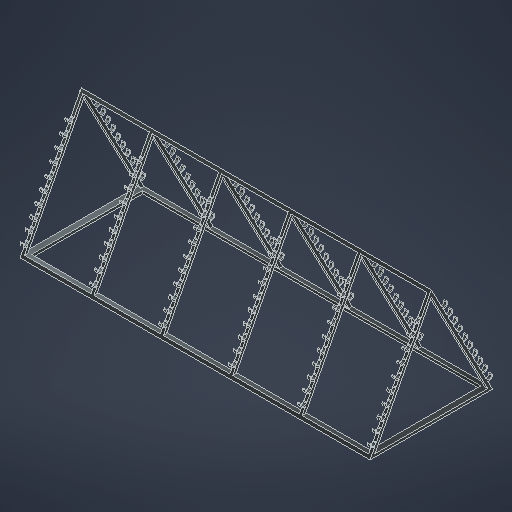
# Autodesk Inventor part: Torre
Saved by Autodesk Inventor 2026.1 (Build 301233020, 233B)
## iProperties
Created: 2025-11-02
Part Number: Torre
Material: Hierro, gris
Document SubType Name: Modeling
Designer: PAVILION
Density: 7.15 g/cm^3
Appearance: Gris hierro
Author: PAVILION
Autodesk Inventor part; units mm, degrees
ref_plane "YZ Plane" through (0, 0, 0) normal (1, 0, 0) x (0, 1, 0)
ref_plane "XZ Plane" through (0, 0, 0) normal (0, 1, 0) x (-1, 0, 0)
ref_plane "XY Plane" through (0, 0, 0) normal (0, 0, 1) x (1, 0, 0)
sketch "Boceto2" plane through (0, 0, 0) normal (1, 0, 0) x (0, 1, 0)
  line L0 (0, 0) -> (2000, 0)
  line L1 (0, 1050) -> (0, -1050)
  line L2 (2000, 0) -> (0, 1050)
  line L3 (2000, 0) -> (0, -1050)
  line L4 (1892.4347, 0) -> (50, 967.2782)
  line L5 (50, 967.2782) -> (50, -967.2782)
  line L6 (50, -967.2782) -> (1892.4347, 0)
  line L7 (200, 945) -> (200, -945)
  line L8 (362, 859.95) -> (362, -859.95)
  line L9 (524, 774.9) -> (524, -774.9)
  line L10 (686, 689.85) -> (686, -689.85)
  line L11 (848, 604.8) -> (848, -604.8)
  line L12 (1010, 519.75) -> (1010, -519.75)
  line L13 (1172, 434.7) -> (1172, -434.7)
  line L14 (1334, 349.65) -> (1334, -349.65)
  line L15 (1496, 264.6) -> (1496, -264.6)
  line L16 (1658, 179.55) -> (1658, -179.55)
  arc A0 (222.9629, 1038.4173) -> (200, 945) centre (211.77, 991.6377) ccw construction
  arc A1 (225.2899, 1048.1428) -> (197.553, 935.304) centre (211.77, 991.6377) ccw
  arc A2 (220.6359, 1028.6918) -> (202.447, 954.696) centre (211.77, 991.6377) ccw
  arc A3 (220.6359, 1028.6918) -> (225.2899, 1048.1428) centre (222.9629, 1038.4173) ccw
  arc A4 (197.553, 935.304) -> (202.447, 954.696) centre (200, 945) ccw
  arc A5 (388.0719, 952.4704) -> (362, 859.95) centre (376.879, 905.6908) ccw construction
  arc A6 (390.3989, 962.1959) -> (358.9066, 850.4405) centre (376.879, 905.6908) ccw
  arc A7 (385.7449, 942.7449) -> (365.0934, 869.4595) centre (376.879, 905.6908) ccw
  arc A8 (385.7449, 942.7449) -> (390.3989, 962.1959) centre (388.0719, 952.4704) ccw
  arc A9 (358.9066, 850.4405) -> (365.0934, 869.4595) centre (362, 859.95) ccw
  arc A10 (524.6943, 764.9241) -> (523.3057, 784.8759) centre (524, 774.9) ccw
  arc A11 (538.8131, 856.3817) -> (548.3419, 873.9658) centre (543.5775, 865.1737) ccw
  arc A12 (538.8131, 856.3817) -> (523.3057, 784.8759) centre (520.6606, 822.8839) ccw
  arc A13 (543.5775, 865.1737) -> (524, 774.9) centre (520.6606, 822.8839) ccw construction
  arc A14 (548.3419, 873.9658) -> (524.6943, 764.9241) centre (520.6606, 822.8839) ccw
  arc A15 (686.078, 679.8503) -> (685.922, 699.8497) centre (686, 689.85) ccw
  arc A16 (695.4303, 774.7651) -> (700.5775, 794.0915) centre (698.0039, 784.4283) ccw
  arc A17 (695.4303, 774.7651) -> (685.922, 699.8497) centre (685.6249, 737.9485) ccw
  arc A18 (698.0039, 784.4283) -> (686, 689.85) centre (685.6249, 737.9485) ccw construction
  arc A19 (700.5775, 794.0915) -> (686.078, 679.8503) centre (685.6249, 737.9485) ccw
  arc A20 (848.9573, 594.8459) -> (847.0427, 614.7541) centre (848, 604.8) ccw
  arc A21 (855.7302, 688.7271) -> (862.2053, 707.6499) centre (858.9678, 698.1885) ccw
  arc A22 (858.9678, 698.1885) -> (848, 604.8) centre (843.3952, 652.6791) ccw construction
  arc A23 (862.2053, 707.6499) -> (848.9573, 594.8459) centre (843.3952, 652.6791) ccw
  arc A24 (855.7302, 688.7271) -> (847.0427, 614.7541) centre (843.3952, 652.6791) ccw
  arc A25 (1010.4664, 509.7609) -> (1009.5336, 529.7391) centre (1010, 519.75) ccw
  arc A26 (1014.5671, 605.284) -> (1018.1422, 624.9619) centre (1016.3547, 615.1229) ccw
  arc A27 (1014.5671, 605.284) -> (1009.5336, 529.7391) centre (1007.7565, 567.7976) ccw
  arc A28 (1016.3547, 615.1229) -> (1010, 519.75) centre (1007.7565, 567.7976) ccw construction
  arc A29 (1018.1422, 624.9619) -> (1010.4664, 509.7609) centre (1007.7565, 567.7976) ccw
  arc A30 (1170.3484, 424.8373) -> (1173.6516, 444.5627) centre (1172, 434.7) ccw
  arc A31 (1185.089, 519.8905) -> (1173.6516, 444.5627) centre (1179.9441, 482.1395) ccw
  arc A32 (1186.4394, 529.7989) -> (1172, 434.7) centre (1179.9441, 482.1395) ccw construction
  arc A33 (1187.7898, 539.7073) -> (1170.3484, 424.8373) centre (1179.9441, 482.1395) ccw
  arc A34 (1185.089, 519.8905) -> (1187.7898, 539.7073) centre (1186.4394, 529.7989) ccw
  arc A35 (1331.7811, 339.8993) -> (1336.2189, 359.4007) centre (1334, 349.65) ccw
  arc A36 (1351.0826, 434.1079) -> (1336.2189, 359.4007) centre (1344.6731, 396.5509) ccw
  arc A37 (1352.7649, 443.9654) -> (1334, 349.65) centre (1344.6731, 396.5509) ccw construction
  arc A38 (1354.4472, 453.8229) -> (1331.7811, 339.8993) centre (1344.6731, 396.5509) ccw
  arc A39 (1351.0826, 434.1079) -> (1354.4472, 453.8229) centre (1352.7649, 443.9654) ccw
  arc A40 (1517.4545, 348.081) -> (1522.6924, 367.383) centre (1520.0734, 357.732) ccw
  arc A41 (1517.4545, 348.081) -> (1498.386, 274.3112) centre (1507.4764, 311.3108) ccw
  arc A42 (1493.614, 254.8888) -> (1498.386, 274.3112) centre (1496, 264.6) ccw
  arc A43 (1520.0734, 357.732) -> (1496, 264.6) centre (1507.4764, 311.3108) ccw construction
  arc A44 (1522.6924, 367.383) -> (1493.614, 254.8888) centre (1507.4764, 311.3108) ccw
  arc A45 (1654.6752, 170.1189) -> (1661.3248, 188.9811) centre (1658, 179.55) ccw
  arc A46 (1683.3502, 261.8465) -> (1661.3248, 188.9811) centre (1673.9925, 224.9135) ccw
  arc A47 (1685.8063, 271.5402) -> (1658, 179.55) centre (1673.9925, 224.9135) ccw construction
  arc A48 (1688.2623, 281.2339) -> (1654.6752, 170.1189) centre (1673.9925, 224.9135) ccw
  arc A49 (1683.3502, 261.8465) -> (1688.2623, 281.2339) centre (1685.8063, 271.5402) ccw
  arc A50 (200, -945) -> (222.9629, -1038.4173) centre (211.77, -991.6377) ccw construction
  arc A51 (197.553, -935.304) -> (225.2899, -1048.1428) centre (211.77, -991.6377) ccw
  arc A52 (202.447, -954.696) -> (220.6359, -1028.6918) centre (211.77, -991.6377) ccw
  arc A53 (225.2899, -1048.1428) -> (220.6359, -1028.6918) centre (222.9629, -1038.4173) ccw
  arc A54 (202.447, -954.696) -> (197.553, -935.304) centre (200, -945) ccw
  arc A55 (365.0934, -869.4595) -> (358.9066, -850.4405) centre (362, -859.95) ccw
  arc A56 (390.3989, -962.1959) -> (385.7449, -942.7449) centre (388.0719, -952.4704) ccw
  arc A57 (365.0934, -869.4595) -> (385.7449, -942.7449) centre (376.879, -905.6908) ccw
  arc A58 (362, -859.95) -> (388.0719, -952.4704) centre (376.879, -905.6908) ccw construction
  arc A59 (358.9066, -850.4405) -> (390.3989, -962.1959) centre (376.879, -905.6908) ccw
  arc A60 (523.3057, -784.8759) -> (524.6943, -764.9241) centre (524, -774.9) ccw
  arc A61 (548.3419, -873.9658) -> (538.8131, -856.3817) centre (543.5775, -865.1737) ccw
  arc A62 (523.3057, -784.8759) -> (538.8131, -856.3817) centre (520.6606, -822.8839) ccw
  arc A63 (524, -774.9) -> (543.5775, -865.1737) centre (520.6606, -822.8839) ccw construction
  arc A64 (524.6943, -764.9241) -> (548.3419, -873.9658) centre (520.6606, -822.8839) ccw
  arc A65 (685.922, -699.8497) -> (686.078, -679.8503) centre (686, -689.85) ccw
  arc A66 (700.5775, -794.0915) -> (695.4303, -774.7651) centre (698.0039, -784.4283) ccw
  arc A67 (686, -689.85) -> (698.0039, -784.4283) centre (685.6249, -737.9485) ccw construction
  arc A68 (686.078, -679.8503) -> (700.5775, -794.0915) centre (685.6249, -737.9485) ccw
  arc A69 (685.922, -699.8497) -> (695.4303, -774.7651) centre (685.6249, -737.9485) ccw
  arc A70 (847.0427, -614.7541) -> (848.9573, -594.8459) centre (848, -604.8) ccw
  arc A71 (862.2053, -707.6499) -> (855.7302, -688.7271) centre (858.9678, -698.1885) ccw
  arc A72 (847.0427, -614.7541) -> (855.7302, -688.7271) centre (843.3952, -652.6791) ccw
  arc A73 (848, -604.8) -> (858.9678, -698.1885) centre (843.3952, -652.6791) ccw construction
  arc A74 (848.9573, -594.8459) -> (862.2053, -707.6499) centre (843.3952, -652.6791) ccw
  arc A75 (1009.5336, -529.7391) -> (1010.4664, -509.7609) centre (1010, -519.75) ccw
  arc A76 (1009.5336, -529.7391) -> (1014.5671, -605.284) centre (1007.7565, -567.7976) ccw
  arc A77 (1010, -519.75) -> (1016.3547, -615.1229) centre (1007.7565, -567.7976) ccw construction
  arc A78 (1010.4664, -509.7609) -> (1018.1422, -624.9619) centre (1007.7565, -567.7976) ccw
  arc A79 (1018.1422, -624.9619) -> (1014.5671, -605.284) centre (1016.3547, -615.1229) ccw
  arc A80 (1173.6516, -444.5627) -> (1170.3484, -424.8373) centre (1172, -434.7) ccw
  arc A81 (1173.6516, -444.5627) -> (1185.089, -519.8905) centre (1179.9441, -482.1395) ccw
  arc A82 (1172, -434.7) -> (1186.4394, -529.7989) centre (1179.9441, -482.1395) ccw construction
  arc A83 (1170.3484, -424.8373) -> (1187.7898, -539.7073) centre (1179.9441, -482.1395) ccw
  arc A84 (1187.7898, -539.7073) -> (1185.089, -519.8905) centre (1186.4394, -529.7989) ccw
  arc A85 (1354.4472, -453.8229) -> (1351.0826, -434.1079) centre (1352.7649, -443.9654) ccw
  arc A86 (1336.2189, -359.4007) -> (1351.0826, -434.1079) centre (1344.6731, -396.5509) ccw
  arc A87 (1336.2189, -359.4007) -> (1331.7811, -339.8993) centre (1334, -349.65) ccw
  arc A88 (1334, -349.65) -> (1352.7649, -443.9654) centre (1344.6731, -396.5509) ccw construction
  arc A89 (1331.7811, -339.8993) -> (1354.4472, -453.8229) centre (1344.6731, -396.5509) ccw
  arc A90 (1498.386, -274.3112) -> (1493.614, -254.8888) centre (1496, -264.6) ccw
  arc A91 (1498.386, -274.3112) -> (1517.4545, -348.081) centre (1507.4764, -311.3108) ccw
  arc A92 (1496, -264.6) -> (1520.0734, -357.732) centre (1507.4764, -311.3108) ccw construction
  arc A93 (1493.614, -254.8888) -> (1522.6924, -367.383) centre (1507.4764, -311.3108) ccw
  arc A94 (1522.6924, -367.383) -> (1517.4545, -348.081) centre (1520.0734, -357.732) ccw
  arc A95 (1688.2623, -281.2339) -> (1683.3502, -261.8465) centre (1685.8063, -271.5402) ccw
  arc A96 (1654.6752, -170.1189) -> (1688.2623, -281.2339) centre (1673.9925, -224.9135) ccw
  arc A97 (1661.3248, -188.9811) -> (1683.3502, -261.8465) centre (1673.9925, -224.9135) ccw
  arc A98 (1658, -179.55) -> (1685.8063, -271.5402) centre (1673.9925, -224.9135) ccw construction
  arc A99 (1661.3248, -188.9811) -> (1654.6752, -170.1189) centre (1658, -179.55) ccw
  point P0 (362, 0)
  point P1 (312.784, 788.7029)
  point P2 (524, 0)
  point P3 (461.0296, 697.0924)
  point P4 (686, 0)
  point P5 (835.0047, 590.2711)
  point P6 (848, 0)
  point P7 (804.8988, 519.75)
  point P8 (788.1671, 504.3238)
  point P9 (1010, 0)
  point P10 (971.3706, 434.7)
  point P11 (1172, 0)
  point P12 (1199.0684, 349.65)
  point P13 (1334, 0)
  point P14 (1280.8287, 264.6)
  point P15 (1496, 0)
  point P16 (1429.0611, 179.55)
  point P17 (1658, 0)
  point P18 (362, -859.95)
  point P19 (524, -774.9)
  point P20 (686, -689.85)
  point P21 (848, -604.8)
  point P22 (1010, -519.75)
  point P23 (1172, -434.7)
  point P24 (1334, -349.65)
  point P25 (1496, -264.6)
  point P26 (1658, -179.55)
  point P27 (312.784, -788.7029)
  point P28 (461.0296, -697.0924)
  point P29 (835.0047, -590.2711)
  point P30 (788.1671, -504.3238)
  point P31 (804.8988, -519.75)
  point P32 (971.3706, -434.7)
  point P33 (1199.0684, -349.65)
  point P34 (1280.8287, -264.6)
  point P35 (1429.0611, -179.55)
  point P36 (1180.854, -430.0517)
  point P37 (1126.9332, -458.3601)
  point P38 (1018.854, -515.1017)
  point P39 (952.4635, -549.9566)
  point P40 (856.854, -600.1517)
  point P41 (787.5887, -636.5159)
  point P42 (694.854, -685.2017)
  point P43 (630.7517, -718.8553)
  point P44 (532.854, -770.2517)
  point P45 (465.1264, -805.8086)
  point P46 (370.854, -855.3017)
  point P47 (325.1098, -879.3173)
  point P48 (208.854, -940.3517)
  point P49 (159.5058, -966.2595)
  point P50 (1342.854, -345.0017)
  point P51 (1292.2078, -371.5909)
  point P52 (1504.854, -259.9517)
  point P53 (1455.1595, -286.0412)
  point P54 (1666.854, -174.9017)
  point P55 (1622.3688, -198.2564)
  point P56 (1622.3688, 198.2564)
  point P57 (1666.854, 174.9017)
  point P58 (1455.1595, 286.0412)
  point P59 (1504.854, 259.9517)
  point P60 (1292.2078, 371.5909)
  point P61 (1342.854, 345.0017)
  point P62 (1126.9332, 458.3601)
  point P63 (1180.854, 430.0517)
  point P64 (952.4635, 549.9566)
  point P65 (1018.854, 515.1017)
  point P66 (787.5887, 636.5159)
  point P67 (856.854, 600.1517)
  point P68 (630.7517, 718.8553)
  point P69 (694.854, 685.2017)
  point P70 (465.1264, 805.8086)
  point P71 (532.854, 770.2517)
  point P72 (325.1098, 879.3173)
  point P73 (370.854, 855.3017)
  point P74 (159.5058, 966.2595)
  point P75 (208.854, 940.3517)
  dimension "d0" = 2000
  dimension "d1" = 2100
  dimension "d5" = 50
  dimension "d6" = 50
  dimension "d7" = 50
  dimension "d8" = 50
  dimension "d11" = 200
  dimension "d69" = 162
  dimension "d70" = 162
  dimension "d71" = 162
  dimension "d72" = 162
  dimension "d73" = 162
  dimension "d74" = 162
  dimension "d75" = 162
  dimension "d76" = 162
  dimension "d77" = 1658
  dimension "d78" = 38.1
  dimension "d79" = 10
  dimension "d80" = 211.77
  dimension "d81" = 38.1
  dimension "d82" = 10
  dimension "d83" = 376.879
  dimension "d84" = 38.1
  dimension "d85" = 10
  dimension "d86" = 38.1
  dimension "d87" = 10
  dimension "d88" = 38.1
  dimension "d89" = 10
  dimension "d90" = 520.6606
  dimension "d91" = 685.6249
  dimension "d92" = 843.3952
  dimension "d93" = 38.1
  dimension "d94" = 10
  dimension "d95" = 1007.7565
  dimension "d96" = 38.1
  dimension "d97" = 10
  dimension "d98" = 1179.9441
  dimension "d99" = 38.1
  dimension "d100" = 10
  dimension "d101" = 1344.6731
  dimension "d102" = 38.1
  dimension "d103" = 10
  dimension "d104" = 173.4764
  dimension "d105" = 38.1
  dimension "d106" = 10
  dimension "d107" = 177.9925
  constraints: 200 point on circle, 100 centre point, 87 symmetric about line, 40 tangent, 30 end point, 12 vertical, 10 midpoint, 9 coincident, 9 vertical alignment, 5 horizontal alignment, 1 horizontal, 1 point on line, 76 other
  measures "d0" distance of L0.start L0.end
  measures "d1" distance of L1.start L1.end
  measures "d5" distance between parallel lines of L1 L5
  measures "d11" distance between parallel lines of L7 L1
  measures "d69" distance between parallel lines of L8 L7
  measures "d70" distance between parallel lines of L9 L8
  measures "d71" distance between parallel lines of L11 L10
  measures "d72" distance between parallel lines of L16 L15
  measures "d73" distance between parallel lines of L10 L9
  measures "d74" distance between parallel lines of L13 L12
  measures "d75" distance between parallel lines of L14 L13
  measures "d76" distance between parallel lines of L15 L14
  measures "d77" distance between parallel lines of L1 L16
  measures "d78" radius of A2
  measures "d79" radius of A3
  measures "d80" horizontal distance of L1.start A0.centre
  measures "d81" radius of A7
  measures "d82" radius of A8
  measures "d83" distance from line of L1 A7.centre
  measures "d84" radius of A12
  measures "d85" radius of A11
  measures "d86" radius of A17
  measures "d87" radius of A16
  measures "d88" radius of A24
  measures "d89" radius of A21
  measures "d90" distance from line of L1 A12.centre
  measures "d91" distance from line of L1 A18.centre
  measures "d92" distance from line of L1 A24.centre
  measures "d93" radius of A27
  measures "d94" radius of A26
  measures "d95" distance from line of L1 A27.centre
  measures "d96" radius of A31
  measures "d97" radius of A34
  measures "d98" distance from line of L1 A31.centre
  measures "d99" radius of A36
  measures "d100" radius of A39
  measures "d101" distance from line of L1 A36.centre
  measures "d102" radius of A41
  measures "d103" radius of A40
  measures "d104" distance from line of L14 A41.centre
  measures "d105" radius of A46
  measures "d106" radius of A49
  measures "d107" distance from line of L15 A48.centre
extrude "Extrusión1" add sketch "Boceto2" along normal mid plane 6000 contours L4 L16 A45 L2 L0 | L0 L3 A99 L16 L6 | L4 L15 A42 L2 A48 A45 L16 | L16 A99 A96 L3 A90 L15 L6 | A45 L16 L2 | L2 A48 A49 A46 A45 | A99 A97 A95 A96 L3 | L3 L16 A99 | L4 L14 A35 L2 A44 A42 L15 | A45 A48 L2 L16 | L15 A90 A93 L3 A87 L14 L6 | L16 L3 A96 A99 | L4 L13 A30 L2 A38 A35 L14 | A42 A44 L2 L15 | L15 L2 A42 | L14 A87 A89 L3 A80 L13 L6 | A90 L3 L15 | L15 L3 A93 A90 | L4 L12 A29 A25 L2 A33 A30 L13 | A35 A38 L2 L14 | L14 L2 A35 | L2 A44 A40 A41 A42 | L13 A80 A83 L3 A75 A78 L12 L6 | A87 L3 L14 | L14 L3 A89 A87 | L3 A90 A91 A94 A93 | L4 L11 A23 A20 L2 A29 L12 | A30 A33 L2 L13 | L13 L2 A30 | L2 A38 A39 A36 A35 | L12 A78 L3 A70 A74 L11 L6 | A80 L3 L13 | L13 L3 A83 A80 | L3 A87 A86 A85 A89 | L4 L10 A19 A15 L2 A23 L11 | A29 L2 L12 | L12 L2 A25 A29 | L2 A33 A34 A31 A30 | L11 A74 L3 A65 A68 L10 L6 | A78 A75 L3 L12 | L12 L3 A78 | L3 A80 A81 A84 A83 | L4 L9 A14 A10 L2 A19 L10 | A23 L2 L11 | L11 L2 A20 A23 | L2 A29 A26 A27 A25 | L10 A68 L3 A60 A64 L9 L6 | A74 A70 L3 L11 | L11 L3 A74 | L3 A75 A76 A79 A78 | L4 L8 A9 L2 A14 L9 | A19 L2 L10 | L10 L2 A15 A19 | L2 A23 A21 A24 A20 | L9 A64 L3 A55 L8 L6 | A68 A65 L3 L10 | L10 L3 A68 | L3 A70 A72 A71 A74 | L4 L7 A4 L2 A6 A9 L8 | A14 L2 L9 | L9 L2 A10 A14 | L2 A19 A16 A17 A15 | L8 A55 A59 L3 A54 L7 L6 | A64 A60 L3 L9 | L9 L3 A64 | L3 A65 A69 A66 A68 | L4 L5 L0 L1 L2 A1 A4 L7 | A9 A6 L2 L8 | L8 L2 A9 | L2 A14 A11 A12 A10 | L7 A54 A51 L3 L1 L0 L5 L6 | A55 L3 L8 | L8 L3 A59 A55 | L3 A60 A62 A61 A64 | A4 A1 L2 L7 | L7 L2 A4 | L2 A6 A8 A7 A9 | A54 L3 L7 | L7 L3 A51 A54 | L3 A55 A57 A56 A59 | L2 A1 A3 A2 A4 | L3 A54 A52 A53 A51
sketch "Boceto3" plane through (0, 0, 0) normal (0, 0, 1) x (1, 0, 0)
  line L0 (2950, 2000) -> (1810, 2000)
  line L1 (1810, 2000) -> (1810, 0)
  line L2 (1810, 0) -> (2950, 0)
  line L3 (2950, 0) -> (2950, 2000)
  line L4 (3000, 50) -> (3000, 1892.4347) projected
  line L5 (3000, 0) -> (-3000, 0) projected
  line L6 (1810, 2000) -> (1760, 2000)
  line L7 (1760, 2000) -> (1760, 0)
  line L8 (1760, 0) -> (1810, 0)
  line L9 (1810, 0) -> (1810, 2000)
  line L10 (3000, 2000) -> (3000, 1666.854) projected
  line L11 (-3000, 2000) -> (3000, 2000) projected
  line L12 (-3000, 1666.854) -> (-3000, 2000) projected
  line L13 (1760, 2000) -> (620, 2000)
  line L14 (620, 2000) -> (620, 0)
  line L15 (620, 0) -> (1760, 0)
  line L16 (1760, 0) -> (1760, 2000)
  line L17 (620, 2000) -> (570, 2000)
  line L18 (570, 2000) -> (570, 0)
  line L19 (570, 0) -> (620, 0)
  line L20 (620, 0) -> (620, 2000)
  line L21 (570, 2000) -> (-570, 2000)
  line L22 (-570, 2000) -> (-570, 0)
  line L23 (-570, 0) -> (570, 0)
  line L24 (570, 0) -> (570, 2000)
  line L25 (-570, 2000) -> (-620, 2000)
  line L26 (-620, 2000) -> (-620, 0)
  line L27 (-620, 0) -> (-570, 0)
  line L28 (-570, 0) -> (-570, 2000)
  line L29 (-620, 2000) -> (-1760, 2000)
  line L30 (-1760, 2000) -> (-1760, 0)
  line L31 (-1760, 0) -> (-620, 0)
  line L32 (-620, 0) -> (-620, 2000)
  line L33 (-1760, 2000) -> (-1810, 2000)
  line L34 (-1810, 2000) -> (-1810, 0)
  line L35 (-1810, 0) -> (-1760, 0)
  line L36 (-1760, 0) -> (-1760, 2000)
  line L37 (-1810, 2000) -> (-2950, 2000)
  line L38 (-2950, 2000) -> (-2950, 0)
  line L39 (-2950, 0) -> (-1810, 0)
  line L40 (-1810, 0) -> (-1810, 2000)
  line L41 (-3000, 1892.4347) -> (-3000, 50) projected
  line L42 (3000, 2000) -> (3000, 0) projected
  line L43 (-3000, 0) -> (-3000, 2000) projected
  line L44 (3000, 2000) -> (-3000, 2000)
  line L45 (-3000, 2000) -> (-3000, 1950)
  line L46 (-3000, 1950) -> (3000, 1950)
  line L47 (3000, 1950) -> (3000, 2000)
  line L48 (-3000, 50) -> (3000, 50) projected
  line L49 (3000, 0) -> (-3000, 0) projected
  line L50 (-3000, 1666.854) -> (3000, 1666.854) projected
  line L51 (-3000, 1504.854) -> (3000, 1504.854) projected
  line L52 (3000, 1622.3688) -> (3000, 1504.854) projected
  line L53 (-3000, 1622.3688) -> (3000, 1622.3688) projected
  line L54 (-3000, 1504.854) -> (-3000, 1622.3688) projected
  line L55 (-3000, 1342.854) -> (3000, 1342.854) projected
  line L56 (3000, 1455.1595) -> (3000, 1342.854) projected
  line L57 (-3000, 1455.1595) -> (3000, 1455.1595) projected
  line L58 (-3000, 1342.854) -> (-3000, 1455.1595) projected
  line L59 (-3000, 1180.854) -> (3000, 1180.854) projected
  line L60 (3000, 1292.2078) -> (3000, 1180.854) projected
  line L61 (-3000, 1292.2078) -> (3000, 1292.2078) projected
  line L62 (-3000, 1180.854) -> (-3000, 1292.2078) projected
  line L63 (-3000, 1018.854) -> (3000, 1018.854) projected
  line L64 (3000, 1126.9332) -> (3000, 1018.854) projected
  line L65 (-3000, 1126.9332) -> (3000, 1126.9332) projected
  line L66 (-3000, 1018.854) -> (-3000, 1126.9332) projected
  line L67 (-3000, 856.854) -> (3000, 856.854) projected
  line L68 (3000, 952.4635) -> (3000, 856.854) projected
  line L69 (-3000, 952.4635) -> (3000, 952.4635) projected
  line L70 (-3000, 856.854) -> (-3000, 952.4635) projected
  line L71 (-3000, 694.854) -> (3000, 694.854) projected
  line L72 (3000, 787.5887) -> (3000, 694.854) projected
  line L73 (-3000, 787.5887) -> (3000, 787.5887) projected
  line L74 (-3000, 694.854) -> (-3000, 787.5887) projected
  line L75 (-3000, 532.854) -> (3000, 532.854) projected
  line L76 (3000, 630.7517) -> (3000, 532.854) projected
  line L77 (-3000, 630.7517) -> (3000, 630.7517) projected
  line L78 (-3000, 532.854) -> (-3000, 630.7517) projected
  line L79 (-3000, 370.854) -> (3000, 370.854) projected
  line L80 (3000, 465.1264) -> (3000, 370.854) projected
  line L81 (-3000, 465.1264) -> (3000, 465.1264) projected
  line L82 (-3000, 370.854) -> (-3000, 465.1264) projected
  line L83 (-3000, 208.854) -> (3000, 208.854) projected
  line L84 (3000, 325.1098) -> (3000, 208.854) projected
  line L85 (-3000, 325.1098) -> (3000, 325.1098) projected
  line L86 (-3000, 208.854) -> (-3000, 325.1098) projected
  line L87 (3000, 159.5058) -> (3000, 0) projected
  line L88 (-3000, 159.5058) -> (3000, 159.5058) projected
  line L89 (-3000, 0) -> (-3000, 159.5058) projected
  point P0 (0, 0)
  point P1 (-3000, 1668.0258)
  point P2 (-1810, 1000)
  point P3 (3000, 167.3998)
  point P4 (-3000, 167.3998)
  point P5 (-2950, 50)
  point P6 (-1810, 50)
  point P7 (-1810, 1950)
  point P8 (-2950, 1950)
  point P9 (-1760, 50)
  point P10 (-620, 50)
  point P11 (-620, 1950)
  point P12 (-1760, 1950)
  point P13 (-570, 50)
  point P14 (570, 50)
  point P15 (570, 1950)
  point P16 (-570, 1950)
  point P17 (620, 50)
  point P18 (1760, 50)
  point P19 (1760, 1950)
  point P20 (620, 1950)
  point P21 (1810, 50)
  point P22 (2950, 50)
  point P23 (2950, 1950)
  point P24 (1810, 1950)
  dimension "d46" = 50
  dimension "d47" = 1140
  dimension "d49" = 50
  dimension "d50" = 1140
  dimension "d51" = 50
  dimension "d52" = 1140
  dimension "d53" = 50
  dimension "d54" = 1140
  dimension "d55" = 50
  dimension "d56" = 1140
  dimension "d57" = 50
  dimension "d58" = 50
  constraints: 80 end point, 20 parallel, 10 horizontal, 10 perpendicular, 1 midpoint, 1 point on line, 9 other
  measures "d46" distance between parallel lines of L4 L3
  measures "d47" distance between parallel lines of L3 L1
  measures "d49" distance of L0.end L6.end
  measures "d50" distance between parallel lines of L16 L14
  measures "d51" distance between parallel lines of L20 L18
  measures "d52" distance between parallel lines of L18 L22
  measures "d53" distance between parallel lines of L22 L26
  measures "d54" distance between parallel lines of L26 L30
  measures "d55" distance from line of L30 point (-1810, 1000)
  measures "d56" distance between parallel lines of L40 L38
  measures "d57" distance between parallel lines of L46 L11
  measures "d58" distance of the line from the sketch origin of L48
extrude "Extrusión2" cut sketch "Boceto3" along normal blind 2000 and the other way blind 2000 contours L3 L50 L1 L46 | L3 L53 L1 L50 | L7 L50 L14 L46 | L3 L51 L1 L53 | L7 L53 L14 L50 | L3 L57 L1 L51 | L7 L51 L14 L53 | L18 L50 L22 L46 | L3 L55 L1 L57 | L7 L57 L14 L51 | L18 L53 L22 L50 | L3 L61 L1 L55 | L7 L55 L14 L57 | L18 L51 L22 L53 | L26 L50 L30 L46 | L3 L59 L1 L61 | L7 L61 L14 L55 | L18 L57 L22 L51 | L26 L53 L30 L50 | L3 L65 L1 L59 | L7 L59 L14 L61 | L18 L55 L22 L57 | L26 L51 L30 L53 | L34 L50 L38 L46 | L3 L63 L1 L65 | L7 L65 L14 L59 | L18 L61 L22 L55 | L26 L57 L30 L51 | L34 L53 L38 L50 | L3 L69 L1 L63 | L7 L63 L14 L65 | L18 L59 L22 L61 | L26 L55 L30 L57 | L34 L51 L38 L53 | L3 L67 L1 L69 | L7 L69 L14 L63 | L18 L65 L22 L59 | L26 L61 L30 L55 | L34 L57 L38 L51 | L3 L73 L1 L67 | L7 L67 L14 L69 | L18 L63 L22 L65 | L26 L59 L30 L61 | L34 L55 L38 L57 | L3 L71 L1 L73 | L7 L73 L14 L67 | L18 L69 L22 L63 | L26 L65 L30 L59 | L34 L61 L38 L55 | L3 L77 L1 L71 | L7 L71 L14 L73 | L18 L67 L22 L69 | L26 L63 L30 L65 | L34 L59 L38 L61 | L3 L75 L1 L77 | L7 L77 L14 L71 | L18 L73 L22 L67 | L26 L69 L30 L63 | L34 L65 L38 L59 | L3 L81 L1 L75 | L7 L75 L14 L77 | L18 L71 L22 L73 | L26 L67 L30 L69 | L34 L63 L38 L65 | L3 L79 L1 L81 | L7 L81 L14 L75 | L18 L77 L22 L71 | L26 L73 L30 L67 | L34 L69 L38 L63 | L3 L85 L1 L79 | L7 L79 L14 L81 | L18 L75 L22 L77 | L26 L71 L30 L73 | L34 L67 L38 L69 | L3 L83 L1 L85 | L7 L85 L14 L79 | L18 L81 L22 L75 | L26 L77 L30 L71 | L34 L73 L38 L67 | L3 L88 L1 L83 | L7 L83 L14 L85 | L18 L79 L22 L81 | L26 L75 L30 L77 | L34 L71 L38 L73 | L3 L48 L1 L88 | L7 L88 L14 L83 | L18 L85 L22 L79 | L26 L81 L30 L75 | L34 L77 L38 L71 | L7 L48 L14 L88 | L18 L83 L22 L85 | L26 L79 L30 L81 | L34 L75 L38 L77 | L18 L88 L22 L83 | L26 L85 L30 L79 | L34 L81 L38 L75 | L18 L48 L22 L88 | L26 L83 L30 L85 | L34 L79 L38 L81 | L26 L88 L30 L83 | L34 L85 L38 L79 | L26 L48 L30 L88 | L34 L83 L38 L85 | L34 L88 L38 L83 | L34 L48 L38 L88
sketch "Boceto4" plane through (-3000, 0, -1050) normal (0, -1, 0) x (1, 0, 0)
  line L0 (0, 0) -> (6000, 0) projected
  line L1 (6000, 2100) -> (6000, 0) projected
  line L2 (6000, 2100) -> (0, 2100) projected
  line L3 (0, 0) -> (0, 2100) projected
  line L4 (5900, 100) -> (100, 100)
  line L5 (100, 100) -> (100, 2000)
  line L6 (100, 2000) -> (5900, 2000)
  line L7 (5900, 2000) -> (5900, 100)
  line L8 (5900, 100) -> (100, 2000) construction
  line L9 (100, 100) -> (5900, 2000) construction
  line L10 (4810, 2017.2782) -> (4810, 2073.75) projected
  line L11 (5900, 100) -> (4810, 100)
  line L12 (4810, 100) -> (4810, 2000)
  line L13 (4810, 2000) -> (5900, 2000)
  line L14 (5900, 2000) -> (5900, 100)
  line L15 (4760, 181.6569) -> (4760, 40.7865) projected
  line L16 (4760, 100) -> (3680, 100)
  line L17 (3680, 100) -> (3680, 2000)
  line L18 (3680, 2000) -> (4760, 2000)
  line L19 (4760, 2000) -> (4760, 100)
  line L20 (3570, 96.5131) -> (3570, -44.3573) projected
  line L21 (2430, 2079.2135) -> (2430, 1927.1823) projected
  line L22 (3570, 96.5131) -> (2430, 96.5131)
  line L23 (2430, 96.5131) -> (2430, 2000)
  line L24 (2430, 2000) -> (3570, 2000)
  line L25 (3570, 2000) -> (3570, 96.5131)
  line L26 (2380, 82.7218) -> (2380, 26.25) projected
  line L27 (1240, 2017.2782) -> (1240, 2073.75) projected
  line L28 (2380, 100) -> (1240, 100)
  line L29 (1240, 100) -> (1240, 2000)
  line L30 (1240, 2000) -> (2380, 2000)
  line L31 (2380, 2000) -> (2380, 100)
  line L32 (100, 2000) -> (1180, 2000)
  line L33 (1180, 2000) -> (1180, 100)
  line L34 (1180, 100) -> (100, 100)
  line L35 (100, 100) -> (100, 2000)
  point P0 (3000, 1050)
  point P1 (4760, 49.5541)
  point P2 (3570, -35.5897)
  point P3 (2430, 2068.1447)
  point P4 (2360, 165.4436)
  point P5 (1280, 1934.5564)
  point P6 (3570, 100)
  point P7 (2430, 100)
  point P8 (3680, 100)
  point P9 (4820, 1934.5564)
  dimension "d63" = 100
  dimension "d64" = 100
  dimension "d65" = 1080
  dimension "d66" = 1080
  constraints: 52 end point, 12 parallel, 12 point on line, 6 horizontal, 6 perpendicular, 2 midpoint
  measures "d63" distance between parallel lines of L0 L4
  measures "d64" distance between parallel lines of L5 L3
  measures "d65" distance between parallel lines of L19 L17
  measures "d66" distance between parallel lines of L33 L5
extrude "Extrusión3" cut sketch "Boceto4" against normal blind 70 contours L4 L12 L6 L7 | L4 L15 L19 L6 L12 | L4 L17 L6 L19 L15 | L4 L25 L6 L17 | L4 L23 L21 L6 L25 | L4 L31 L6 L21 L23 | L4 L29 L6 L31 | L4 L33 L6 L29 | L4 L5 L6 L33
sketch "Boceto5" plane through (-3000, 0, 0) normal (-1, 0, 0) x (0, 0, 1)
  line L0 (-20, 1961.9048) -> (20, 1961.9048)
  line L1 (20, 1961.9048) -> (20, 1892.4347)
  line L2 (20, 1892.4347) -> (-20, 1892.4347)
  line L3 (-20, 1892.4347) -> (-20, 1961.9048)
  line L4 (0, 2000) -> (-174.9017, 1666.854) projected
  line L5 (174.9017, 1666.854) -> (0, 2000) projected
  point P0 (0, 0)
  point P1 (0, 1892.4347)
  dimension "d108" = 40
  constraints: 8 end point, 2 parallel, 2 point on line, 1 horizontal, 1 midpoint, 1 perpendicular
  measures "d108" distance of L0.start L0.end
extrude "Extrusión4" add sketch "Boceto5" along normal blind 10 contours L0 L1 L2 L3
